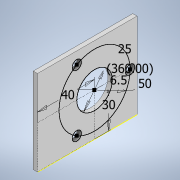
# Autodesk Inventor part: motorbracket
Saved by Autodesk Inventor 2021.5 (Build 255421000, 421)
## iProperties
Created: 2024-11-18
Part Number: motorbracket
Material: Generic
Document SubType Name: Modeling
Designer: email
Density: 1 g/cm^3
Appearance: Default
Author: email
Autodesk Inventor part; units mm, degrees
ref_plane "YZ Plane" through (0, 0, 0) normal (1, 0, 0) x (0, 1, 0)
ref_plane "XZ Plane" through (0, 0, 0) normal (0, 1, 0) x (-1, 0, 0)
ref_plane "XY Plane" through (0, 0, 0) normal (0, 0, 1) x (1, 0, 0)
sketch "Sketch1" plane through (0, 0, 0) normal (0, 1, 0) x (-1, 0, 0)
  line L0 (0, 0) -> (-3, 0)
  line L1 (-3, 0) -> (-3, -70)
  line L2 (-3, -70) -> (0, -70)
  line L3 (0, -70) -> (0, 0)
  line L4 (0, -3) -> (0, 0)
  dimension "d0" = 3
  dimension "d1" = 70
  constraints: 10 end point, 2 parallel, 1 horizontal, 1 perpendicular
  measures "d0" distance between parallel lines of L3 L1
  measures "d1" distance of L0.end L1.end
extrude "Extrusion1" add sketch "Sketch1" along normal blind 60
sketch "Sketch2" plane through (3, 0, -3) normal (1, 0, 0) x (0, 0, -1)
  line L0 (67, 0) -> (-3, 0) projected
  line L1 (-3, 0) -> (37, 0) construction
  line L2 (37, 0) -> (37, 30) construction
  line L3 (37, 30) -> (-3, 30) construction
  line L4 (-3, 30) -> (-3, 0) construction
  circle A0 centre (37, 30) radius 25
  line L5 (37, 30) -> (62, 30) construction
  circle A1 centre (62, 30) radius 3.25
  circle A2 centre (24.5, 51.6506) radius 3.25
  circle A3 centre (24.5, 8.3494) radius 3.25
  circle A4 centre (37, 30) radius 12.5
  dimension "d8" = 50
  dimension "d6" = 30
  dimension "d7" = 40
  dimension "d9" = 6.5
  dimension "d12" = 360
  dimension "d36" = 25
  constraints: 10 end point, 4 centre point, 3 coincident, 2 horizontal, 2 parallel, 1 horizontal alignment, 1 perpendicular, 9 other
  measures "d6" distance of L1.end L2.end
  measures "d7" distance of L2.end L3.end
  measures "d9" diameter of A1
  measures "d36" diameter of A4
hole "Hole1" at (3, 8.3494, -27.5) at (3, 51.6506, -27.5) at (3, 30, -65) direction (-1, 0, 0) diameter 6.5 depth 10
extrude "Extrusion2" cut sketch "Sketch2" against normal blind 50 contours A4
body "Solid1"
